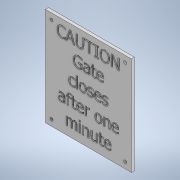
# Autodesk Inventor part: warningSignV2
Saved by Autodesk Inventor 2021.2 (Build 252289000, 289)
## iProperties
Created: 2020-11-24
Part Number: warningSignV2
Material: Generic
Document SubType Name: Modeling
Designer: robst
Density: 1 g/cm^3
Appearance: Default
Author: robst
Autodesk Inventor part; units mm, degrees
ref_plane "YZ Plane" through (0, 0, 0) normal (1, 0, 0) x (0, 1, 0)
ref_plane "XZ Plane" through (0, 0, 0) normal (0, 1, 0) x (-1, 0, 0)
ref_plane "XY Plane" through (0, 0, 0) normal (0, 0, 1) x (1, 0, 0)
sketch "Sketch4" plane through (0, 0, 0) normal (0, 0, 1) x (1, 0, 0)
  line L0 (-88.9, -101.6) -> (88.9, -101.6)
  line L1 (88.9, -101.6) -> (88.9, 101.6)
  line L2 (88.9, 101.6) -> (-88.9, 101.6)
  line L3 (-88.9, 101.6) -> (-88.9, -101.6)
  line L4 (-88.9, -101.6) -> (88.9, 101.6) construction
  line L5 (88.9, -101.6) -> (-88.9, 101.6) construction
  point P0 (0, 0)
  dimension "d12" = 203.2
  dimension "d13" = 177.8
  constraints: 12 end point, 2 midpoint, 2 parallel, 1 horizontal, 1 perpendicular
  measures "d12" distance of L2.end L0.start
  measures "d13" distance of L0.start L0.end
extrude "Extrusion2" add sketch "Sketch4" against normal blind 6.35
sketch "Sketch5" plane through (0, 0, 0) normal (0, 0, 1) x (1, 0, 0)
  line L0 (-88.9, -101.6) -> (-88.9, 101.6) construction
  line L1 (-88.9, 67.31) -> (88.9, 67.31) construction
  line L2 (88.9, 101.6) -> (88.9, -101.6) construction
  line L3 (88.9, 101.6) -> (-88.9, 101.6) construction
  spline S0 degree 2 poles (-54.5935, 66.9024) (-56.8165, 66.9024) (-60.5771, 68.403) (-61.948, 69.9035) knots 0 0 0 1 2 2 2
  spline S1 degree 2 poles (-61.948, 69.9035) (-63.3189, 71.3855) (-64.8194, 75.8316) (-64.8194, 78.7215) knots 0 0 0 1 2 2 2
  spline S2 degree 2 poles (-64.8194, 78.7215) (-64.8194, 81.5929) (-63.3559, 85.8536) (-61.9665, 87.4283) knots 0 0 0 1 2 2 2
  spline S3 degree 2 poles (-61.9665, 87.4283) (-60.5957, 88.9659) (-56.8536, 90.5776) (-54.538, 90.5776) knots 0 0 0 1 2 2 2
  spline S4 degree 2 poles (-54.538, 90.5776) (-53.3894, 90.5776) (-51.3702, 90.2441) (-50.518, 89.9847) knots 0 0 0 1 2 2 2
  spline S5 degree 2 poles (-50.518, 89.9847) (-49.777, 89.7439) (-48.2394, 89.0585) (-47.4799, 88.6509) knots 0 0 0 1 2 2 2
  line L4 (-47.4799, 88.6509) -> (-47.4799, 84.983)
  line L5 (-47.4799, 84.983) -> (-47.7207, 84.983)
  spline S6 degree 2 poles (-47.7207, 84.983) (-48.1283, 85.3535) (-49.388, 86.3909) (-50.2957, 86.8911) knots 0 0 0 1 2 2 2
  spline S7 degree 2 poles (-50.2957, 86.8911) (-51.1664, 87.3727) (-53.2227, 87.984) (-54.5565, 87.984) knots 0 0 0 1 2 2 2
  spline S8 degree 2 poles (-54.5565, 87.984) (-56.02, 87.984) (-58.632, 86.7799) (-59.6138, 85.6313) knots 0 0 0 1 2 2 2
  spline S9 degree 2 poles (-59.6138, 85.6313) (-60.5771, 84.4643) (-61.6516, 80.926) (-61.6516, 78.7215) knots 0 0 0 1 2 2 2
  spline S10 degree 2 poles (-61.6516, 78.7215) (-61.6516, 76.3688) (-60.5216, 72.9787) (-59.5397, 71.8116) knots 0 0 0 1 2 2 2
  spline S11 degree 2 poles (-59.5397, 71.8116) (-58.5764, 70.6816) (-56.0014, 69.533) (-54.5565, 69.533) knots 0 0 0 1 2 2 2
  spline S12 degree 2 poles (-54.5565, 69.533) (-53.2412, 69.533) (-50.9997, 70.1814) (-50.129, 70.663) knots 0 0 0 1 2 2 2
  spline S13 degree 2 poles (-50.129, 70.663) (-49.2953, 71.1447) (-48.0542, 72.1451) (-47.7022, 72.497) knots 0 0 0 1 2 2 2
  line L6 (-47.7022, 72.497) -> (-47.4799, 72.497)
  line L7 (-47.4799, 72.497) -> (-47.4799, 68.8661)
  spline S14 degree 2 poles (-47.4799, 68.8661) (-48.2394, 68.5141) (-49.5732, 67.8658) (-50.518, 67.5694) knots 0 0 0 1 2 2 2
  spline S15 degree 2 poles (-50.518, 67.5694) (-51.5184, 67.2359) (-53.2227, 66.9024) (-54.5935, 66.9024) knots 0 0 0 1 2 2 2
  line L8 (-47.1094, 67.31) -> (-39.4029, 90.17)
  line L9 (-39.4029, 90.17) -> (-35.6609, 90.17)
  line L10 (-35.6609, 90.17) -> (-27.9544, 67.31)
  line L11 (-27.9544, 67.31) -> (-31.1593, 67.31)
  line L12 (-31.1593, 67.31) -> (-33.2341, 73.7012)
  line L13 (-33.2341, 73.7012) -> (-41.9594, 73.7012)
  line L14 (-41.9594, 73.7012) -> (-44.0342, 67.31)
  line L15 (-44.0342, 67.31) -> (-47.1094, 67.31)
  line L16 (-34.0677, 76.2947) -> (-37.606, 87.0578)
  line L17 (-37.606, 87.0578) -> (-41.1258, 76.2947)
  line L18 (-41.1258, 76.2947) -> (-34.0677, 76.2947)
  spline S16 degree 2 poles (-17.5062, 66.8283) (-19.5255, 66.8283) (-22.5265, 67.8843) (-23.5825, 68.9402) knots 0 0 0 1 2 2 2
  spline S17 degree 2 poles (-23.5825, 68.9402) (-24.7866, 70.1258) (-25.7684, 73.4603) (-25.7684, 75.9057) knots 0 0 0 1 2 2 2
  line L19 (-25.7684, 75.9057) -> (-25.7684, 90.17)
  line L20 (-25.7684, 90.17) -> (-22.7303, 90.17)
  line L21 (-22.7303, 90.17) -> (-22.7303, 75.9057)
  spline S18 degree 2 poles (-22.7303, 75.9057) (-22.7303, 74.3125) (-22.3228, 72.1636) (-21.7485, 71.2929) knots 0 0 0 1 2 2 2
  spline S19 degree 2 poles (-21.7485, 71.2929) (-21.1372, 70.3666) (-19.0253, 69.4219) (-17.5062, 69.4219) knots 0 0 0 1 2 2 2
  spline S20 degree 2 poles (-17.5062, 69.4219) (-16.0798, 69.4219) (-13.8568, 70.3666) (-13.2455, 71.2929) knots 0 0 0 1 2 2 2
  spline S21 degree 2 poles (-13.2455, 71.2929) (-12.6712, 72.1636) (-12.2636, 74.294) (-12.2636, 75.8316) knots 0 0 0 1 2 2 2
  line L22 (-12.2636, 75.8316) -> (-12.2636, 90.17)
  line L23 (-12.2636, 90.17) -> (-9.2255, 90.17)
  line L24 (-9.2255, 90.17) -> (-9.2255, 75.9057)
  spline S22 degree 2 poles (-9.2255, 75.9057) (-9.2255, 73.5159) (-10.1888, 70.1073) (-11.4115, 68.9402) knots 0 0 0 1 2 2 2
  spline S23 degree 2 poles (-11.4115, 68.9402) (-12.5045, 67.8658) (-15.3944, 66.8283) (-17.5062, 66.8283) knots 0 0 0 1 2 2 2
  line L25 (0.4631, 67.31) -> (0.4631, 87.4653)
  line L26 (0.4631, 87.4653) -> (-7.2063, 87.4653)
  line L27 (-7.2063, 87.4653) -> (-7.2063, 90.17)
  line L28 (-7.2063, 90.17) -> (11.1706, 90.17)
  line L29 (11.1706, 90.17) -> (11.1706, 87.4653)
  line L30 (11.1706, 87.4653) -> (3.5012, 87.4653)
  line L31 (3.5012, 87.4653) -> (3.5012, 67.31)
  line L32 (3.5012, 67.31) -> (0.4631, 67.31)
  line L33 (21.4706, 67.31) -> (12.6156, 67.31)
  line L34 (12.6156, 67.31) -> (12.6156, 69.6442)
  line L35 (12.6156, 69.6442) -> (15.5241, 69.6442)
  line L36 (15.5241, 69.6442) -> (15.5241, 87.8358)
  line L37 (15.5241, 87.8358) -> (12.6156, 87.8358)
  line L38 (12.6156, 87.8358) -> (12.6156, 90.17)
  line L39 (12.6156, 90.17) -> (21.4706, 90.17)
  line L40 (21.4706, 90.17) -> (21.4706, 87.8358)
  line L41 (21.4706, 87.8358) -> (18.5622, 87.8358)
  line L42 (18.5622, 87.8358) -> (18.5622, 69.6442)
  line L43 (18.5622, 69.6442) -> (21.4706, 69.6442)
  line L44 (21.4706, 69.6442) -> (21.4706, 67.31)
  spline S24 degree 2 poles (41.4036, 87.558) (42.7004, 86.0389) (44.1454, 81.5929) (44.1454, 78.74) knots 0 0 0 1 2 2 2
  spline S25 degree 2 poles (44.1454, 78.74) (44.1454, 75.9612) (42.7375, 71.4596) (41.4036, 69.9406) knots 0 0 0 1 2 2 2
  spline S26 degree 2 poles (41.4036, 69.9406) (39.9957, 68.3474) (36.2722, 66.8283) (34.0306, 66.8283) knots 0 0 0 1 2 2 2
  spline S27 degree 2 poles (34.0306, 66.8283) (31.715, 66.8283) (28.01, 68.403) (26.6577, 69.9406) knots 0 0 0 1 2 2 2
  spline S28 degree 2 poles (26.6577, 69.9406) (25.3424, 71.4596) (23.9345, 75.9242) (23.9345, 78.74) knots 0 0 0 1 2 2 2
  spline S29 degree 2 poles (23.9345, 78.74) (23.9345, 81.6114) (25.3609, 85.9833) (26.6762, 87.558) knots 0 0 0 1 2 2 2
  spline S30 degree 2 poles (26.6762, 87.558) (28.01, 89.077) (31.7335, 90.6517) (34.0306, 90.6517) knots 0 0 0 1 2 2 2
  spline S31 degree 2 poles (34.0306, 90.6517) (36.3648, 90.6517) (40.1069, 89.0214) (41.4036, 87.558) knots 0 0 0 1 2 2 2
  spline S32 degree 2 poles (40.9776, 78.74) (40.9776, 81.0001) (39.9957, 84.5013) (39.1065, 85.6499) knots 0 0 0 1 2 2 2
  spline S33 degree 2 poles (39.1065, 85.6499) (38.1988, 86.8355) (35.6423, 88.0211) (34.0492, 88.0211) knots 0 0 0 1 2 2 2
  spline S34 degree 2 poles (34.0492, 88.0211) (32.4004, 88.0211) (29.9181, 86.8725) (28.9733, 85.6499) knots 0 0 0 1 2 2 2
  spline S35 degree 2 poles (28.9733, 85.6499) (28.0656, 84.4828) (27.1023, 80.963) (27.1023, 78.74) knots 0 0 0 1 2 2 2
  spline S36 degree 2 poles (27.1023, 78.74) (27.1023, 74.2384) (30.8814, 69.4589) (34.0492, 69.4589) knots 0 0 0 1 2 2 2
  spline S37 degree 2 poles (34.0492, 69.4589) (37.217, 69.4589) (40.9776, 74.2384) (40.9776, 78.74) knots 0 0 0 1 2 2 2
  line L45 (63.8376, 67.31) -> (60.4289, 67.31)
  line L46 (60.4289, 67.31) -> (50.3142, 87.0207)
  line L47 (50.3142, 87.0207) -> (50.3142, 67.31)
  line L48 (50.3142, 67.31) -> (47.4799, 67.31)
  line L49 (47.4799, 67.31) -> (47.4799, 90.17)
  line L50 (47.4799, 90.17) -> (51.7962, 90.17)
  line L51 (51.7962, 90.17) -> (61.0032, 72.071)
  line L52 (61.0032, 72.071) -> (61.0032, 90.17)
  line L53 (61.0032, 90.17) -> (63.8376, 90.17)
  line L54 (63.8376, 90.17) -> (63.8376, 67.31)
  spline S38 degree 2 poles (-20.3869, 29.1894) (-22.8137, 29.1894) (-26.8336, 30.6714) (-28.2786, 32.172) knots 0 0 0 1 2 2 2
  spline S39 degree 2 poles (-28.2786, 32.172) (-29.7236, 33.691) (-31.2611, 38.1741) (-31.2611, 41.0826) knots 0 0 0 1 2 2 2
  spline S40 degree 2 poles (-31.2611, 41.0826) (-31.2611, 43.8428) (-29.705, 48.2147) (-28.2601, 49.7708) knots 0 0 0 1 2 2 2
  spline S41 degree 2 poles (-28.2601, 49.7708) (-26.8707, 51.2714) (-22.7952, 52.9016) (-20.3684, 52.9016) knots 0 0 0 1 2 2 2
  spline S42 degree 2 poles (-20.3684, 52.9016) (-19.2013, 52.9016) (-17.0894, 52.5681) (-16.1261, 52.2717) knots 0 0 0 1 2 2 2
  spline S43 degree 2 poles (-16.1261, 52.2717) (-15.3481, 52.0494) (-13.4585, 51.2343) (-12.8842, 50.9379) knots 0 0 0 1 2 2 2
  line L55 (-12.8842, 50.9379) -> (-12.8842, 47.2699)
  line L56 (-12.8842, 47.2699) -> (-13.1436, 47.2699)
  spline S44 degree 2 poles (-13.1436, 47.2699) (-13.7179, 47.7701) (-14.922, 48.6779) (-16.0335, 49.1966) knots 0 0 0 1 2 2 2
  spline S45 degree 2 poles (-16.0335, 49.1966) (-16.9597, 49.6597) (-19.3495, 50.271) (-20.7203, 50.271) knots 0 0 0 1 2 2 2
  spline S46 degree 2 poles (-20.7203, 50.271) (-24.0178, 50.271) (-28.0933, 45.3063) (-28.0933, 41.1752) knots 0 0 0 1 2 2 2
  spline S47 degree 2 poles (-28.0933, 41.1752) (-28.0933, 38.8781) (-27.0189, 35.4324) (-26, 34.2468) knots 0 0 0 1 2 2 2
  spline S48 degree 2 poles (-26, 34.2468) (-25.0182, 33.0612) (-22.2394, 31.82) (-20.498, 31.82) knots 0 0 0 1 2 2 2
  spline S49 degree 2 poles (-20.498, 31.82) (-19.2198, 31.82) (-16.6633, 32.1905) (-15.7927, 32.561) knots 0 0 0 1 2 2 2
  line L57 (-15.7927, 32.561) -> (-15.7927, 38.4705)
  line L58 (-15.7927, 38.4705) -> (-21.0908, 38.4705)
  line L59 (-21.0908, 38.4705) -> (-21.0908, 41.1381)
  line L60 (-21.0908, 41.1381) -> (-12.7916, 41.1381)
  line L61 (-12.7916, 41.1381) -> (-12.7916, 31.1531)
  spline S50 degree 2 poles (-12.7916, 31.1531) (-13.3659, 30.8937) (-15.3295, 30.0972) (-16.1632, 29.8563) knots 0 0 0 1 2 2 2
  spline S51 degree 2 poles (-16.1632, 29.8563) (-17.2932, 29.5229) (-19.1087, 29.1894) (-20.3869, 29.1894) knots 0 0 0 1 2 2 2
  spline S52 degree 2 poles (0.3612, 31.4495) (0.0093, 31.1901) (-1.1763, 30.2639) (-1.7321, 29.986) knots 0 0 0 1 2 2 2
  spline S53 degree 2 poles (-1.7321, 29.986) (-2.4916, 29.5785) (-3.9181, 29.1524) (-5.2148, 29.1524) knots 0 0 0 1 2 2 2
  spline S54 degree 2 poles (-5.2148, 29.1524) (-6.2708, 29.1524) (-8.1788, 29.949) (-8.9013, 30.6714) knots 0 0 0 1 2 2 2
  spline S55 degree 2 poles (-8.9013, 30.6714) (-9.5867, 31.3754) (-10.4204, 33.4502) (-10.4204, 34.5988) knots 0 0 0 1 2 2 2
  spline S56 degree 2 poles (-10.4204, 34.5988) (-10.4204, 36.3772) (-8.9198, 38.8966) (-7.2896, 39.6191) knots 0 0 0 1 2 2 2
  spline S57 degree 2 poles (-7.2896, 39.6191) (-5.8447, 40.286) (-1.9173, 40.7862) (0.3612, 40.9158) knots 0 0 0 1 2 2 2
  line L62 (0.3612, 40.9158) -> (0.3612, 41.4716)
  spline S58 degree 2 poles (0.3612, 41.4716) (0.3612, 42.4719) (-0.2501, 43.7131) (-0.8058, 44.0651) knots 0 0 0 1 2 2 2
  spline S59 degree 2 poles (-0.8058, 44.0651) (-1.3616, 44.4171) (-2.9548, 44.6394) (-3.8069, 44.6394) knots 0 0 0 1 2 2 2
  spline S60 degree 2 poles (-3.8069, 44.6394) (-4.8073, 44.6394) (-7.5119, 44.0466) (-8.8643, 43.4723) knots 0 0 0 1 2 2 2
  line L63 (-8.8643, 43.4723) -> (-9.031, 43.4723)
  line L64 (-9.031, 43.4723) -> (-9.031, 46.4178)
  spline S61 degree 2 poles (-9.031, 46.4178) (-8.2344, 46.6401) (-5.2519, 47.1958) (-3.7884, 47.1958) knots 0 0 0 1 2 2 2
  spline S62 degree 2 poles (-3.7884, 47.1958) (-2.01, 47.1958) (0.4168, 46.6401) (1.3801, 45.9176) knots 0 0 0 1 2 2 2
  spline S63 degree 2 poles (1.3801, 45.9176) (2.3249, 45.2137) (3.2512, 42.9721) (3.2512, 41.3604) knots 0 0 0 1 2 2 2
  line L65 (3.2512, 41.3604) -> (3.2512, 29.634)
  line L66 (3.2512, 29.634) -> (0.3612, 29.634)
  line L67 (0.3612, 29.634) -> (0.3612, 31.4495)
  line L68 (0.3612, 33.8578) -> (0.3612, 38.6187)
  spline S64 degree 2 poles (0.3612, 38.6187) (-0.6762, 38.5261) (-3.8069, 38.2112) (-4.7887, 37.9148) knots 0 0 0 1 2 2 2
  spline S65 degree 2 poles (-4.7887, 37.9148) (-5.9373, 37.5628) (-7.4378, 36.0993) (-7.4378, 34.8025) knots 0 0 0 1 2 2 2
  spline S66 degree 2 poles (-7.4378, 34.8025) (-7.4378, 33.3205) (-5.7706, 31.82) (-4.1774, 31.82) knots 0 0 0 1 2 2 2
  spline S67 degree 2 poles (-4.1774, 31.82) (-2.8251, 31.82) (-0.6021, 32.9871) (0.3612, 33.8578) knots 0 0 0 1 2 2 2
  spline S68 degree 2 poles (12.4952, 29.3006) (10.1425, 29.3006) (7.4934, 31.9867) (7.4934, 34.8952) knots 0 0 0 1 2 2 2
  line L69 (7.4934, 34.8952) -> (7.4934, 44.3985)
  line L70 (7.4934, 44.3985) -> (5.5483, 44.3985)
  line L71 (5.5483, 44.3985) -> (5.5483, 46.7883)
  line L72 (5.5483, 46.7883) -> (7.4934, 46.7883)
  line L73 (7.4934, 46.7883) -> (7.4934, 51.716)
  line L74 (7.4934, 51.716) -> (10.3833, 51.716)
  line L75 (10.3833, 51.716) -> (10.3833, 46.7883)
  line L76 (10.3833, 46.7883) -> (15.7, 46.7883)
  line L77 (15.7, 46.7883) -> (15.7, 44.3985)
  line L78 (15.7, 44.3985) -> (10.3833, 44.3985)
  line L79 (10.3833, 44.3985) -> (10.3833, 36.229)
  spline S69 degree 2 poles (10.3833, 36.229) (10.3833, 34.9322) (10.476, 33.5058) (10.7909, 32.8944) knots 0 0 0 1 2 2 2
  spline S70 degree 2 poles (10.7909, 32.8944) (11.0502, 32.3572) (12.2173, 31.82) (13.2177, 31.82) knots 0 0 0 1 2 2 2
  spline S71 degree 2 poles (13.2177, 31.82) (13.9216, 31.82) (15.2369, 32.2461) (15.5333, 32.3757) knots 0 0 0 1 2 2 2
  line L80 (15.5333, 32.3757) -> (15.7, 32.3757)
  line L81 (15.7, 32.3757) -> (15.7, 29.7822)
  spline S72 degree 2 poles (15.7, 29.7822) (14.8849, 29.5599) (13.2177, 29.3006) (12.4952, 29.3006) knots 0 0 0 1 2 2 2
  spline S73 degree 2 poles (25.2775, 29.245) (21.165, 29.245) (16.6448, 33.8578) (16.6448, 38.1185) knots 0 0 0 1 2 2 2
  spline S74 degree 2 poles (16.6448, 38.1185) (16.6448, 42.3052) (21.0353, 47.2699) (24.5736, 47.2699) knots 0 0 0 1 2 2 2
  spline S75 degree 2 poles (24.5736, 47.2699) (26.1667, 47.2699) (28.6306, 46.3437) (29.5383, 45.3619) knots 0 0 0 1 2 2 2
  spline S76 degree 2 poles (29.5383, 45.3619) (30.4646, 44.38) (31.4464, 41.5457) (31.4464, 39.4894) knots 0 0 0 1 2 2 2
  line L82 (31.4464, 39.4894) -> (31.4464, 37.9148)
  line L83 (31.4464, 37.9148) -> (19.5718, 37.9148)
  spline S77 degree 2 poles (19.5718, 37.9148) (19.5718, 34.9322) (22.5729, 31.7644) (25.2405, 31.7644) knots 0 0 0 1 2 2 2
  spline S78 degree 2 poles (25.2405, 31.7644) (26.1853, 31.7644) (28.0192, 32.1905) (28.7603, 32.5239) knots 0 0 0 1 2 2 2
  spline S79 degree 2 poles (28.7603, 32.5239) (29.5383, 32.8944) (30.6128, 33.5428) (30.9647, 33.8392) knots 0 0 0 1 2 2 2
  line L84 (30.9647, 33.8392) -> (31.1315, 33.8392)
  line L85 (31.1315, 33.8392) -> (31.1315, 30.69)
  spline S80 degree 2 poles (31.1315, 30.69) (30.6313, 30.4862) (29.1122, 29.8934) (28.5194, 29.7267) knots 0 0 0 1 2 2 2
  spline S81 degree 2 poles (28.5194, 29.7267) (27.6858, 29.4858) (26.3149, 29.245) (25.2775, 29.245) knots 0 0 0 1 2 2 2
  spline S82 degree 2 poles (28.6306, 40.1192) (28.5935, 41.2863) (28.1119, 42.9906) (27.6487, 43.5649) knots 0 0 0 1 2 2 2
  spline S83 degree 2 poles (27.6487, 43.5649) (27.1486, 44.2133) (25.5739, 44.8987) (24.4068, 44.8987) knots 0 0 0 1 2 2 2
  spline S84 degree 2 poles (24.4068, 44.8987) (23.2583, 44.8987) (21.6466, 44.2133) (20.9797, 43.5464) knots 0 0 0 1 2 2 2
  spline S85 degree 2 poles (20.9797, 43.5464) (20.3313, 42.861) (19.6644, 41.2122) (19.5718, 40.1192) knots 0 0 0 1 2 2 2
  line L86 (19.5718, 40.1192) -> (28.6306, 40.1192)
  spline S86 degree 2 poles (-32.7617, -9.0423) (-34.5401, -9.0423) (-37.4856, -7.9493) (-38.5415, -6.8378) knots 0 0 0 1 2 2 2
  spline S87 degree 2 poles (-38.5415, -6.8378) (-39.5974, -5.7448) (-40.7645, -2.3733) (-40.7645, -0.1132) knots 0 0 0 1 2 2 2
  spline S88 degree 2 poles (-40.7645, -0.1132) (-40.7645, 2.1469) (-39.5604, 5.4443) (-38.5415, 6.5559) knots 0 0 0 1 2 2 2
  spline S89 degree 2 poles (-38.5415, 6.5559) (-37.5226, 7.6859) (-34.503, 8.89) (-32.7617, 8.89) knots 0 0 0 1 2 2 2
  spline S90 degree 2 poles (-32.7617, 8.89) (-31.3538, 8.89) (-28.7232, 8.0934) (-27.7043, 7.5747) knots 0 0 0 1 2 2 2
  line L87 (-27.7043, 7.5747) -> (-27.7043, 4.3328)
  line L88 (-27.7043, 4.3328) -> (-27.871, 4.3328)
  spline S91 degree 2 poles (-27.871, 4.3328) (-28.186, 4.5922) (-29.1493, 5.2591) (-29.8347, 5.6111) knots 0 0 0 1 2 2 2
  spline S92 degree 2 poles (-29.8347, 5.6111) (-30.446, 5.9075) (-32.0762, 6.3706) (-32.8173, 6.3706) knots 0 0 0 1 2 2 2
  spline S93 degree 2 poles (-32.8173, 6.3706) (-35.0588, 6.3706) (-37.782, 2.9805) (-37.782, -0.1132) knots 0 0 0 1 2 2 2
  spline S94 degree 2 poles (-37.782, -0.1132) (-37.782, -3.1328) (-35.1514, -6.5229) (-32.8173, -6.5229) knots 0 0 0 1 2 2 2
  spline S95 degree 2 poles (-32.8173, -6.5229) (-31.4093, -6.5229) (-28.8529, -5.3558) (-27.871, -4.4481) knots 0 0 0 1 2 2 2
  line L89 (-27.871, -4.4481) -> (-27.7043, -4.4481)
  line L90 (-27.7043, -4.4481) -> (-27.7043, -7.69)
  spline S96 degree 2 poles (-27.7043, -7.69) (-28.1304, -7.8937) (-29.4272, -8.468) (-29.9459, -8.5977) knots 0 0 0 1 2 2 2
  spline S97 degree 2 poles (-29.9459, -8.5977) (-30.6869, -8.82) (-31.8539, -9.0423) (-32.7617, -9.0423) knots 0 0 0 1 2 2 2
  line L91 (-22.1283, -8.6533) -> (-25.0182, -8.6533)
  line L92 (-25.0182, -8.6533) -> (-25.0182, 15.2256)
  line L93 (-25.0182, 15.2256) -> (-22.1283, 15.2256)
  line L94 (-22.1283, 15.2256) -> (-22.1283, -8.6533)
  spline S98 degree 2 poles (-3.7884, -0.0761) (-3.7884, -4.411) (-7.9565, -9.1349) (-11.4393, -9.1349) knots 0 0 0 1 2 2 2
  spline S99 degree 2 poles (-11.4393, -9.1349) (-15.0146, -9.1349) (-19.1087, -4.2628) (-19.1087, -0.0761) knots 0 0 0 1 2 2 2
  spline S100 degree 2 poles (-19.1087, -0.0761) (-19.1087, 4.2217) (-14.8849, 8.9826) (-11.4393, 8.9826) knots 0 0 0 1 2 2 2
  spline S101 degree 2 poles (-11.4393, 8.9826) (-7.9565, 8.9826) (-3.7884, 4.2402) (-3.7884, -0.0761) knots 0 0 0 1 2 2 2
  spline S102 degree 2 poles (-6.7709, -0.0761) (-6.7709, 3.2584) (-9.1977, 6.5003) (-11.4393, 6.5003) knots 0 0 0 1 2 2 2
  spline S103 degree 2 poles (-11.4393, 6.5003) (-13.6808, 6.5003) (-16.1261, 3.2584) (-16.1261, -0.0761) knots 0 0 0 1 2 2 2
  spline S104 degree 2 poles (-16.1261, -0.0761) (-16.1261, -3.318) (-13.6808, -6.6526) (-11.4393, -6.6526) knots 0 0 0 1 2 2 2
  spline S105 degree 2 poles (-11.4393, -6.6526) (-9.2162, -6.6526) (-6.7709, -3.3736) (-6.7709, -0.0761) knots 0 0 0 1 2 2 2
  spline S106 degree 2 poles (3.8069, -9.0608) (2.0841, -9.0608) (-0.8985, -8.1346) (-1.8803, -7.6159) knots 0 0 0 1 2 2 2
  line L95 (-1.8803, -7.6159) -> (-1.8803, -4.374)
  line L96 (-1.8803, -4.374) -> (-1.7321, -4.374)
  spline S107 degree 2 poles (-1.7321, -4.374) (-1.3616, -4.6704) (-0.3612, -5.3743) (0.4724, -5.7634) knots 0 0 0 1 2 2 2
  spline S108 degree 2 poles (0.4724, -5.7634) (1.1949, -6.1153) (2.9733, -6.634) (3.9181, -6.634) knots 0 0 0 1 2 2 2
  spline S109 degree 2 poles (3.9181, -6.634) (4.6035, -6.634) (6.1781, -6.3191) (6.5486, -6.0598) knots 0 0 0 1 2 2 2
  spline S110 degree 2 poles (6.5486, -6.0598) (7.0859, -5.7078) (7.5675, -4.9112) (7.5675, -4.0961) knots 0 0 0 1 2 2 2
  spline S111 degree 2 poles (7.5675, -4.0961) (7.5675, -3.0772) (6.456, -2.0213) (5.0296, -1.6693) knots 0 0 0 1 2 2 2
  spline S112 degree 2 poles (5.0296, -1.6693) (4.4738, -1.5396) (2.6954, -1.1691) (1.9359, -0.9653) knots 0 0 0 1 2 2 2
  spline S113 degree 2 poles (1.9359, -0.9653) (-0.0278, -0.3911) (-1.8062, 1.9801) (-1.8062, 3.6659) knots 0 0 0 1 2 2 2
  spline S114 degree 2 poles (-1.8062, 3.6659) (-1.8062, 6.0001) (1.695, 8.9085) (4.585, 8.9085) knots 0 0 0 1 2 2 2
  spline S115 degree 2 poles (4.585, 8.9085) (6.0114, 8.9085) (8.9013, 8.2046) (9.8832, 7.6674) knots 0 0 0 1 2 2 2
  line L97 (9.8832, 7.6674) -> (9.8832, 4.5737)
  line L98 (9.8832, 4.5737) -> (9.735, 4.5737)
  spline S116 degree 2 poles (9.735, 4.5737) (8.6234, 5.4629) (5.9188, 6.4818) (4.5294, 6.4818) knots 0 0 0 1 2 2 2
  spline S117 degree 2 poles (4.5294, 6.4818) (3.103, 6.4818) (1.1393, 5.2776) (1.1393, 4.0735) knots 0 0 0 1 2 2 2
  spline S118 degree 2 poles (1.1393, 4.0735) (1.1393, 2.9805) (2.3064, 1.9246) (3.6031, 1.5911) knots 0 0 0 1 2 2 2
  spline S119 degree 2 poles (3.6031, 1.5911) (4.233, 1.4244) (5.8262, 1.0909) (6.6968, 0.8872) knots 0 0 0 1 2 2 2
  spline S120 degree 2 poles (6.6968, 0.8872) (8.5864, 0.4055) (10.513, -1.799) (10.513, -3.7071) knots 0 0 0 1 2 2 2
  spline S121 degree 2 poles (10.513, -3.7071) (10.513, -4.8186) (9.6423, -6.7822) (8.7902, -7.5047) knots 0 0 0 1 2 2 2
  spline S122 degree 2 poles (8.7902, -7.5047) (7.8824, -8.2642) (5.5668, -9.0608) (3.8069, -9.0608) knots 0 0 0 1 2 2 2
  spline S123 degree 2 poles (20.6462, -9.0423) (16.5337, -9.0423) (12.0135, -4.4295) (12.0135, -0.1688) knots 0 0 0 1 2 2 2
  spline S124 degree 2 poles (12.0135, -0.1688) (12.0135, 4.0179) (16.404, 8.9826) (19.9423, 8.9826) knots 0 0 0 1 2 2 2
  spline S125 degree 2 poles (19.9423, 8.9826) (21.5355, 8.9826) (23.9993, 8.0564) (24.907, 7.0746) knots 0 0 0 1 2 2 2
  spline S126 degree 2 poles (24.907, 7.0746) (25.8333, 6.0927) (26.8151, 3.2584) (26.8151, 1.2021) knots 0 0 0 1 2 2 2
  line L99 (26.8151, 1.2021) -> (26.8151, -0.3725)
  line L100 (26.8151, -0.3725) -> (14.9405, -0.3725)
  spline S127 degree 2 poles (14.9405, -0.3725) (14.9405, -3.3551) (17.9416, -6.5229) (20.6092, -6.5229) knots 0 0 0 1 2 2 2
  spline S128 degree 2 poles (20.6092, -6.5229) (21.554, -6.5229) (23.388, -6.0968) (24.129, -5.7634) knots 0 0 0 1 2 2 2
  spline S129 degree 2 poles (24.129, -5.7634) (24.907, -5.3929) (25.9815, -4.7445) (26.3335, -4.4481) knots 0 0 0 1 2 2 2
  line L101 (26.3335, -4.4481) -> (26.5002, -4.4481)
  line L102 (26.5002, -4.4481) -> (26.5002, -7.5973)
  spline S130 degree 2 poles (26.5002, -7.5973) (26, -7.8011) (24.4809, -8.3939) (23.8881, -8.5606) knots 0 0 0 1 2 2 2
  spline S131 degree 2 poles (23.8881, -8.5606) (23.0545, -8.8015) (21.6837, -9.0423) (20.6462, -9.0423) knots 0 0 0 1 2 2 2
  spline S132 degree 2 poles (23.9993, 1.8319) (23.9622, 2.999) (23.4806, 4.7033) (23.0175, 5.2776) knots 0 0 0 1 2 2 2
  spline S133 degree 2 poles (23.0175, 5.2776) (22.5173, 5.926) (20.9427, 6.6114) (19.7756, 6.6114) knots 0 0 0 1 2 2 2
  spline S134 degree 2 poles (19.7756, 6.6114) (18.627, 6.6114) (17.0153, 5.926) (16.3484, 5.2591) knots 0 0 0 1 2 2 2
  spline S135 degree 2 poles (16.3484, 5.2591) (15.7, 4.5737) (15.0331, 2.9249) (14.9405, 1.8319) knots 0 0 0 1 2 2 2
  line L103 (14.9405, 1.8319) -> (23.9993, 1.8319)
  spline S136 degree 2 poles (34.3734, -9.0608) (32.6505, -9.0608) (29.668, -8.1346) (28.6862, -7.6159) knots 0 0 0 1 2 2 2
  line L104 (28.6862, -7.6159) -> (28.6862, -4.374)
  line L105 (28.6862, -4.374) -> (28.8344, -4.374)
  spline S137 degree 2 poles (28.8344, -4.374) (29.2049, -4.6704) (30.2052, -5.3743) (31.0388, -5.7634) knots 0 0 0 1 2 2 2
  spline S138 degree 2 poles (31.0388, -5.7634) (31.7613, -6.1153) (33.5397, -6.634) (34.4845, -6.634) knots 0 0 0 1 2 2 2
  spline S139 degree 2 poles (34.4845, -6.634) (35.1699, -6.634) (36.7446, -6.3191) (37.1151, -6.0598) knots 0 0 0 1 2 2 2
  spline S140 degree 2 poles (37.1151, -6.0598) (37.6523, -5.7078) (38.134, -4.9112) (38.134, -4.0961) knots 0 0 0 1 2 2 2
  spline S141 degree 2 poles (38.134, -4.0961) (38.134, -3.0772) (37.0225, -2.0213) (35.596, -1.6693) knots 0 0 0 1 2 2 2
  spline S142 degree 2 poles (35.596, -1.6693) (35.0403, -1.5396) (33.2619, -1.1691) (32.5023, -0.9653) knots 0 0 0 1 2 2 2
  spline S143 degree 2 poles (32.5023, -0.9653) (30.5387, -0.3911) (28.7603, 1.9801) (28.7603, 3.6659) knots 0 0 0 1 2 2 2
  spline S144 degree 2 poles (28.7603, 3.6659) (28.7603, 6.0001) (32.2615, 8.9085) (35.1514, 8.9085) knots 0 0 0 1 2 2 2
  spline S145 degree 2 poles (35.1514, 8.9085) (36.5779, 8.9085) (39.4678, 8.2046) (40.4496, 7.6674) knots 0 0 0 1 2 2 2
  line L106 (40.4496, 7.6674) -> (40.4496, 4.5737)
  line L107 (40.4496, 4.5737) -> (40.3014, 4.5737)
  spline S146 degree 2 poles (40.3014, 4.5737) (39.1899, 5.4629) (36.4852, 6.4818) (35.0958, 6.4818) knots 0 0 0 1 2 2 2
  spline S147 degree 2 poles (35.0958, 6.4818) (33.6694, 6.4818) (31.7057, 5.2776) (31.7057, 4.0735) knots 0 0 0 1 2 2 2
  spline S148 degree 2 poles (31.7057, 4.0735) (31.7057, 2.9805) (32.8728, 1.9246) (34.1696, 1.5911) knots 0 0 0 1 2 2 2
  spline S149 degree 2 poles (34.1696, 1.5911) (34.7994, 1.4244) (36.3926, 1.0909) (37.2633, 0.8872) knots 0 0 0 1 2 2 2
  spline S150 degree 2 poles (37.2633, 0.8872) (39.1528, 0.4055) (41.0795, -1.799) (41.0795, -3.7071) knots 0 0 0 1 2 2 2
  spline S151 degree 2 poles (41.0795, -3.7071) (41.0795, -4.8186) (40.2088, -6.7822) (39.3566, -7.5047) knots 0 0 0 1 2 2 2
  spline S152 degree 2 poles (39.3566, -7.5047) (38.4489, -8.2642) (36.1333, -9.0608) (34.3734, -9.0608) knots 0 0 0 1 2 2 2
  spline S153 degree 2 poles (-51.2775, -45.2733) (-51.6295, -45.5327) (-52.8151, -46.4589) (-53.3709, -46.7368) knots 0 0 0 1 2 2 2
  spline S154 degree 2 poles (-53.3709, -46.7368) (-54.1304, -47.1444) (-55.5568, -47.5704) (-56.8536, -47.5704) knots 0 0 0 1 2 2 2
  spline S155 degree 2 poles (-56.8536, -47.5704) (-57.9095, -47.5704) (-59.8176, -46.7738) (-60.5401, -46.0514) knots 0 0 0 1 2 2 2
  spline S156 degree 2 poles (-60.5401, -46.0514) (-61.2255, -45.3474) (-62.0592, -43.2726) (-62.0592, -42.124) knots 0 0 0 1 2 2 2
  spline S157 degree 2 poles (-62.0592, -42.124) (-62.0592, -40.3456) (-60.5586, -37.8262) (-58.9284, -37.1037) knots 0 0 0 1 2 2 2
  spline S158 degree 2 poles (-58.9284, -37.1037) (-57.4834, -36.4368) (-53.5561, -35.9367) (-51.2775, -35.807) knots 0 0 0 1 2 2 2
  line L108 (-51.2775, -35.807) -> (-51.2775, -35.2512)
  spline S159 degree 2 poles (-51.2775, -35.2512) (-51.2775, -34.2509) (-51.8889, -33.0097) (-52.4446, -32.6577) knots 0 0 0 1 2 2 2
  spline S160 degree 2 poles (-52.4446, -32.6577) (-53.0004, -32.3057) (-54.5935, -32.0834) (-55.4457, -32.0834) knots 0 0 0 1 2 2 2
  spline S161 degree 2 poles (-55.4457, -32.0834) (-56.446, -32.0834) (-59.1507, -32.6762) (-60.503, -33.2505) knots 0 0 0 1 2 2 2
  line L109 (-60.503, -33.2505) -> (-60.6698, -33.2505)
  line L110 (-60.6698, -33.2505) -> (-60.6698, -30.305)
  spline S162 degree 2 poles (-60.6698, -30.305) (-59.8732, -30.0827) (-56.8906, -29.527) (-55.4272, -29.527) knots 0 0 0 1 2 2 2
  spline S163 degree 2 poles (-55.4272, -29.527) (-53.6487, -29.527) (-51.222, -30.0827) (-50.2587, -30.8052) knots 0 0 0 1 2 2 2
  spline S164 degree 2 poles (-50.2587, -30.8052) (-49.3139, -31.5091) (-48.3876, -33.7507) (-48.3876, -35.3624) knots 0 0 0 1 2 2 2
  line L111 (-48.3876, -35.3624) -> (-48.3876, -47.0888)
  line L112 (-48.3876, -47.0888) -> (-51.2775, -47.0888)
  line L113 (-51.2775, -47.0888) -> (-51.2775, -45.2733)
  line L114 (-51.2775, -42.865) -> (-51.2775, -38.1041)
  spline S165 degree 2 poles (-51.2775, -38.1041) (-52.3149, -38.1967) (-55.4457, -38.5116) (-56.4275, -38.808) knots 0 0 0 1 2 2 2
  spline S166 degree 2 poles (-56.4275, -38.808) (-57.5761, -39.16) (-59.0766, -40.6235) (-59.0766, -41.9203) knots 0 0 0 1 2 2 2
  spline S167 degree 2 poles (-59.0766, -41.9203) (-59.0766, -43.4023) (-57.4093, -44.9028) (-55.8162, -44.9028) knots 0 0 0 1 2 2 2
  spline S168 degree 2 poles (-55.8162, -44.9028) (-54.4639, -44.9028) (-52.2408, -43.7357) (-51.2775, -42.865) knots 0 0 0 1 2 2 2
  line L115 (-35.3089, -25.9887) -> (-35.4571, -25.9887)
  spline S169 degree 2 poles (-35.4571, -25.9887) (-35.8461, -25.8405) (-37.2911, -25.5811) (-37.8653, -25.5811) knots 0 0 0 1 2 2 2
  spline S170 degree 2 poles (-37.8653, -25.5811) (-39.6808, -25.5811) (-41.2369, -27.2113) (-41.2369, -29.3602) knots 0 0 0 1 2 2 2
  line L116 (-41.2369, -29.3602) -> (-41.2369, -29.9345)
  line L117 (-41.2369, -29.9345) -> (-36.4574, -29.9345)
  line L118 (-36.4574, -29.9345) -> (-36.4574, -32.3243)
  line L119 (-36.4574, -32.3243) -> (-41.1443, -32.3243)
  line L120 (-41.1443, -32.3243) -> (-41.1443, -47.0888)
  line L121 (-41.1443, -47.0888) -> (-44.0342, -47.0888)
  line L122 (-44.0342, -47.0888) -> (-44.0342, -32.3243)
  line L123 (-44.0342, -32.3243) -> (-45.9793, -32.3243)
  line L124 (-45.9793, -32.3243) -> (-45.9793, -29.9345)
  line L125 (-45.9793, -29.9345) -> (-44.0342, -29.9345)
  line L126 (-44.0342, -29.9345) -> (-44.0342, -29.3602)
  spline S171 degree 2 poles (-44.0342, -29.3602) (-44.0342, -26.2851) (-41.0517, -23.0617) (-38.2729, -23.0617) knots 0 0 0 1 2 2 2
  spline S172 degree 2 poles (-38.2729, -23.0617) (-37.4763, -23.0617) (-35.9387, -23.2284) (-35.3089, -23.3396) knots 0 0 0 1 2 2 2
  line L127 (-35.3089, -23.3396) -> (-35.3089, -25.9887)
  spline S173 degree 2 poles (-28.4731, -47.4222) (-30.8258, -47.4222) (-33.4749, -44.7361) (-33.4749, -41.8276) knots 0 0 0 1 2 2 2
  line L128 (-33.4749, -41.8276) -> (-33.4749, -32.3243)
  line L129 (-33.4749, -32.3243) -> (-35.42, -32.3243)
  line L130 (-35.42, -32.3243) -> (-35.42, -29.9345)
  line L131 (-35.42, -29.9345) -> (-33.4749, -29.9345)
  line L132 (-33.4749, -29.9345) -> (-33.4749, -25.0068)
  line L133 (-33.4749, -25.0068) -> (-30.585, -25.0068)
  line L134 (-30.585, -25.0068) -> (-30.585, -29.9345)
  line L135 (-30.585, -29.9345) -> (-25.2683, -29.9345)
  line L136 (-25.2683, -29.9345) -> (-25.2683, -32.3243)
  line L137 (-25.2683, -32.3243) -> (-30.585, -32.3243)
  line L138 (-30.585, -32.3243) -> (-30.585, -40.4938)
  spline S174 degree 2 poles (-30.585, -40.4938) (-30.585, -41.7906) (-30.4923, -43.217) (-30.1774, -43.8284) knots 0 0 0 1 2 2 2
  spline S175 degree 2 poles (-30.1774, -43.8284) (-29.9181, -44.3656) (-28.751, -44.9028) (-27.7506, -44.9028) knots 0 0 0 1 2 2 2
  spline S176 degree 2 poles (-27.7506, -44.9028) (-27.0467, -44.9028) (-25.7314, -44.4767) (-25.435, -44.3471) knots 0 0 0 1 2 2 2
  line L139 (-25.435, -44.3471) -> (-25.2683, -44.3471)
  line L140 (-25.2683, -44.3471) -> (-25.2683, -46.9406)
  spline S177 degree 2 poles (-25.2683, -46.9406) (-26.0834, -47.1629) (-27.7506, -47.4222) (-28.4731, -47.4222) knots 0 0 0 1 2 2 2
  spline S178 degree 2 poles (-15.6908, -47.4778) (-19.8034, -47.4778) (-24.3235, -42.865) (-24.3235, -38.6043) knots 0 0 0 1 2 2 2
  spline S179 degree 2 poles (-24.3235, -38.6043) (-24.3235, -34.4176) (-19.933, -29.4529) (-16.3947, -29.4529) knots 0 0 0 1 2 2 2
  spline S180 degree 2 poles (-16.3947, -29.4529) (-14.8016, -29.4529) (-12.3377, -30.3791) (-11.43, -31.3609) knots 0 0 0 1 2 2 2
  spline S181 degree 2 poles (-11.43, -31.3609) (-10.5037, -32.3428) (-9.5219, -35.1771) (-9.5219, -37.2334) knots 0 0 0 1 2 2 2
  line L141 (-9.5219, -37.2334) -> (-9.5219, -38.808)
  line L142 (-9.5219, -38.808) -> (-21.3965, -38.808)
  spline S182 degree 2 poles (-21.3965, -38.808) (-21.3965, -41.7906) (-18.3954, -44.9584) (-15.7278, -44.9584) knots 0 0 0 1 2 2 2
  spline S183 degree 2 poles (-15.7278, -44.9584) (-14.783, -44.9584) (-12.9491, -44.5323) (-12.2081, -44.1989) knots 0 0 0 1 2 2 2
  spline S184 degree 2 poles (-12.2081, -44.1989) (-11.43, -43.8284) (-10.3555, -43.18) (-10.0036, -42.8836) knots 0 0 0 1 2 2 2
  line L143 (-10.0036, -42.8836) -> (-9.8368, -42.8836)
  line L144 (-9.8368, -42.8836) -> (-9.8368, -46.0328)
  spline S185 degree 2 poles (-9.8368, -46.0328) (-10.337, -46.2366) (-11.8561, -46.8294) (-12.4489, -46.9961) knots 0 0 0 1 2 2 2
  spline S186 degree 2 poles (-12.4489, -46.9961) (-13.2825, -47.237) (-14.6534, -47.4778) (-15.6908, -47.4778) knots 0 0 0 1 2 2 2
  spline S187 degree 2 poles (-12.3377, -36.6036) (-12.3748, -35.4365) (-12.8564, -33.7322) (-13.3196, -33.1579) knots 0 0 0 1 2 2 2
  spline S188 degree 2 poles (-13.3196, -33.1579) (-13.8197, -32.5095) (-15.3944, -31.8241) (-16.5615, -31.8241) knots 0 0 0 1 2 2 2
  spline S189 degree 2 poles (-16.5615, -31.8241) (-17.71, -31.8241) (-19.3217, -32.5095) (-19.9886, -33.1764) knots 0 0 0 1 2 2 2
  spline S190 degree 2 poles (-19.9886, -33.1764) (-20.637, -33.8618) (-21.3039, -35.5106) (-21.3965, -36.6036) knots 0 0 0 1 2 2 2
  line L145 (-21.3965, -36.6036) -> (-12.3377, -36.6036)
  line L146 (2.5009, -33.0282) -> (2.3527, -33.0282)
  spline S191 degree 2 poles (2.3527, -33.0282) (2.0192, -32.9356) (1.2968, -32.8985) (0.7966, -32.8985) knots 0 0 0 1 2 2 2
  spline S192 degree 2 poles (0.7966, -32.8985) (-0.3705, -32.8985) (-2.6676, -33.9174) (-3.705, -34.9178) knots 0 0 0 1 2 2 2
  line L147 (-3.705, -34.9178) -> (-3.705, -47.0888)
  line L148 (-3.705, -47.0888) -> (-6.5949, -47.0888)
  line L149 (-6.5949, -47.0888) -> (-6.5949, -29.9345)
  line L150 (-6.5949, -29.9345) -> (-3.705, -29.9345)
  line L151 (-3.705, -29.9345) -> (-3.705, -32.491)
  spline S193 degree 2 poles (-3.705, -32.491) (-2.1304, -31.0831) (0.2223, -29.9345) (1.3338, -29.9345) knots 0 0 0 1 2 2 2
  spline S194 degree 2 poles (1.3338, -29.9345) (1.7784, -29.9345) (2.223, -29.9716) (2.5009, -30.0271) knots 0 0 0 1 2 2 2
  line L152 (2.5009, -30.0271) -> (2.5009, -33.0282)
  spline S195 degree 2 poles (28.6584, -38.5116) (28.6584, -42.8465) (24.4902, -47.5704) (21.0075, -47.5704) knots 0 0 0 1 2 2 2
  spline S196 degree 2 poles (21.0075, -47.5704) (17.4321, -47.5704) (13.3381, -42.6983) (13.3381, -38.5116) knots 0 0 0 1 2 2 2
  spline S197 degree 2 poles (13.3381, -38.5116) (13.3381, -34.2138) (17.5618, -29.4529) (21.0075, -29.4529) knots 0 0 0 1 2 2 2
  spline S198 degree 2 poles (21.0075, -29.4529) (24.4902, -29.4529) (28.6584, -34.1953) (28.6584, -38.5116) knots 0 0 0 1 2 2 2
  spline S199 degree 2 poles (25.6758, -38.5116) (25.6758, -35.1771) (23.249, -31.9352) (21.0075, -31.9352) knots 0 0 0 1 2 2 2
  spline S200 degree 2 poles (21.0075, -31.9352) (18.7659, -31.9352) (16.3206, -35.1771) (16.3206, -38.5116) knots 0 0 0 1 2 2 2
  spline S201 degree 2 poles (16.3206, -38.5116) (16.3206, -41.7535) (18.7659, -45.0881) (21.0075, -45.0881) knots 0 0 0 1 2 2 2
  spline S202 degree 2 poles (21.0075, -45.0881) (23.2305, -45.0881) (25.6758, -41.8091) (25.6758, -38.5116) knots 0 0 0 1 2 2 2
  line L153 (45.0901, -47.0888) -> (42.2002, -47.0888)
  line L154 (42.2002, -47.0888) -> (42.2002, -37.3075)
  spline S203 degree 2 poles (42.2002, -37.3075) (42.2002, -36.1219) (41.9779, -34.0841) (41.6445, -33.4728) knots 0 0 0 1 2 2 2
  spline S204 degree 2 poles (41.6445, -33.4728) (41.2925, -32.8244) (40.0328, -32.1946) (38.9583, -32.1946) knots 0 0 0 1 2 2 2
  spline S205 degree 2 poles (38.9583, -32.1946) (37.8839, -32.1946) (35.6053, -33.3431) (34.5123, -34.2694) knots 0 0 0 1 2 2 2
  line L155 (34.5123, -34.2694) -> (34.5123, -47.0888)
  line L156 (34.5123, -47.0888) -> (31.6224, -47.0888)
  line L157 (31.6224, -47.0888) -> (31.6224, -29.9345)
  line L158 (31.6224, -29.9345) -> (34.5123, -29.9345)
  line L159 (34.5123, -29.9345) -> (34.5123, -31.8426)
  spline S206 degree 2 poles (34.5123, -31.8426) (35.8091, -30.6755) (38.31, -29.4529) (39.7179, -29.4529) knots 0 0 0 1 2 2 2
  spline S207 degree 2 poles (39.7179, -29.4529) (42.2373, -29.4529) (45.0901, -32.7874) (45.0901, -35.9552) knots 0 0 0 1 2 2 2
  line L160 (45.0901, -35.9552) -> (45.0901, -47.0888)
  spline S208 degree 2 poles (56.5942, -47.4778) (52.4817, -47.4778) (47.9615, -42.865) (47.9615, -38.6043) knots 0 0 0 1 2 2 2
  spline S209 degree 2 poles (47.9615, -38.6043) (47.9615, -34.4176) (52.352, -29.4529) (55.8903, -29.4529) knots 0 0 0 1 2 2 2
  spline S210 degree 2 poles (55.8903, -29.4529) (57.4835, -29.4529) (59.9473, -30.3791) (60.855, -31.3609) knots 0 0 0 1 2 2 2
  spline S211 degree 2 poles (60.855, -31.3609) (61.7813, -32.3428) (62.7631, -35.1771) (62.7631, -37.2334) knots 0 0 0 1 2 2 2
  line L161 (62.7631, -37.2334) -> (62.7631, -38.808)
  line L162 (62.7631, -38.808) -> (50.8885, -38.808)
  spline S212 degree 2 poles (50.8885, -38.808) (50.8885, -41.7906) (53.8896, -44.9584) (56.5572, -44.9584) knots 0 0 0 1 2 2 2
  spline S213 degree 2 poles (56.5572, -44.9584) (57.502, -44.9584) (59.336, -44.5323) (60.077, -44.1989) knots 0 0 0 1 2 2 2
  spline S214 degree 2 poles (60.077, -44.1989) (60.855, -43.8284) (61.9295, -43.18) (62.2815, -42.8836) knots 0 0 0 1 2 2 2
  line L163 (62.2815, -42.8836) -> (62.4482, -42.8836)
  line L164 (62.4482, -42.8836) -> (62.4482, -46.0328)
  spline S215 degree 2 poles (62.4482, -46.0328) (61.948, -46.2366) (60.4289, -46.8294) (59.8361, -46.9961) knots 0 0 0 1 2 2 2
  spline S216 degree 2 poles (59.8361, -46.9961) (59.0025, -47.237) (57.6317, -47.4778) (56.5942, -47.4778) knots 0 0 0 1 2 2 2
  spline S217 degree 2 poles (59.9473, -36.6036) (59.9102, -35.4365) (59.4286, -33.7322) (58.9655, -33.1579) knots 0 0 0 1 2 2 2
  spline S218 degree 2 poles (58.9655, -33.1579) (58.4653, -32.5095) (56.8906, -31.8241) (55.7236, -31.8241) knots 0 0 0 1 2 2 2
  spline S219 degree 2 poles (55.7236, -31.8241) (54.575, -31.8241) (52.9633, -32.5095) (52.2964, -33.1764) knots 0 0 0 1 2 2 2
  spline S220 degree 2 poles (52.2964, -33.1764) (51.648, -33.8618) (50.9811, -35.5106) (50.8885, -36.6036) knots 0 0 0 1 2 2 2
  line L165 (50.8885, -36.6036) -> (59.9473, -36.6036)
  line L166 (-26.3057, -84.5054) -> (-26.3057, -74.5759)
  spline S221 degree 2 poles (-26.3057, -74.5759) (-26.3057, -73.3903) (-26.4909, -71.3711) (-26.7873, -70.8153) knots 0 0 0 1 2 2 2
  spline S222 degree 2 poles (-26.7873, -70.8153) (-27.0837, -70.204) (-28.2138, -69.6112) (-29.1956, -69.6112) knots 0 0 0 1 2 2 2
  spline S223 degree 2 poles (-29.1956, -69.6112) (-30.0848, -69.6112) (-32.1226, -70.7042) (-33.197, -71.7416) knots 0 0 0 1 2 2 2
  spline S224 degree 2 poles (-33.197, -71.7416) (-33.1785, -72.0009) (-33.1414, -72.7234) (-33.1414, -73.2051) knots 0 0 0 1 2 2 2
  line L167 (-33.1414, -73.2051) -> (-33.1414, -84.5054)
  line L168 (-33.1414, -84.5054) -> (-36.0314, -84.5054)
  line L169 (-36.0314, -84.5054) -> (-36.0314, -74.5759)
  spline S225 degree 2 poles (-36.0314, -74.5759) (-36.0314, -73.3903) (-36.2166, -71.3711) (-36.513, -70.8153) knots 0 0 0 1 2 2 2
  spline S226 degree 2 poles (-36.513, -70.8153) (-36.8094, -70.204) (-37.9394, -69.6112) (-38.9213, -69.6112) knots 0 0 0 1 2 2 2
  spline S227 degree 2 poles (-38.9213, -69.6112) (-39.8475, -69.6112) (-41.9038, -70.7783) (-42.8671, -71.686) knots 0 0 0 1 2 2 2
  line L170 (-42.8671, -71.686) -> (-42.8671, -84.5054)
  line L171 (-42.8671, -84.5054) -> (-45.7571, -84.5054)
  line L172 (-45.7571, -84.5054) -> (-45.7571, -67.3511)
  line L173 (-45.7571, -67.3511) -> (-42.8671, -67.3511)
  line L174 (-42.8671, -67.3511) -> (-42.8671, -69.2407)
  spline S228 degree 2 poles (-42.8671, -69.2407) (-41.7371, -68.1107) (-39.5141, -66.8695) (-38.1803, -66.8695) knots 0 0 0 1 2 2 2
  spline S229 degree 2 poles (-38.1803, -66.8695) (-36.6612, -66.8695) (-34.3085, -68.2589) (-33.6972, -69.8335) knots 0 0 0 1 2 2 2
  spline S230 degree 2 poles (-33.6972, -69.8335) (-32.3819, -68.37) (-29.8995, -66.8695) (-28.4546, -66.8695) knots 0 0 0 1 2 2 2
  spline S231 degree 2 poles (-28.4546, -66.8695) (-27.3431, -66.8695) (-25.5276, -67.5549) (-24.8607, -68.333) knots 0 0 0 1 2 2 2
  spline S232 degree 2 poles (-24.8607, -68.333) (-24.1753, -69.111) (-23.4158, -71.4452) (-23.4158, -73.2051) knots 0 0 0 1 2 2 2
  line L175 (-23.4158, -73.2051) -> (-23.4158, -84.5054)
  line L176 (-23.4158, -84.5054) -> (-26.3057, -84.5054)
  line L177 (-16.4133, -84.5054) -> (-19.3032, -84.5054)
  line L178 (-19.3032, -84.5054) -> (-19.3032, -67.3511)
  line L179 (-19.3032, -67.3511) -> (-16.4133, -67.3511)
  line L180 (-16.4133, -67.3511) -> (-16.4133, -84.5054)
  line L181 (-16.2095, -64.4983) -> (-19.4884, -64.4983)
  line L182 (-19.4884, -64.4983) -> (-19.4884, -61.4972)
  line L183 (-19.4884, -61.4972) -> (-16.2095, -61.4972)
  line L184 (-16.2095, -61.4972) -> (-16.2095, -64.4983)
  line L185 (1.2968, -84.5054) -> (-1.5932, -84.5054)
  line L186 (-1.5932, -84.5054) -> (-1.5932, -74.7241)
  spline S233 degree 2 poles (-1.5932, -74.7241) (-1.5932, -73.5385) (-1.8155, -71.5008) (-2.1489, -70.8894) knots 0 0 0 1 2 2 2
  spline S234 degree 2 poles (-2.1489, -70.8894) (-2.5009, -70.2411) (-3.7606, -69.6112) (-4.8351, -69.6112) knots 0 0 0 1 2 2 2
  spline S235 degree 2 poles (-4.8351, -69.6112) (-5.9095, -69.6112) (-8.1881, -70.7598) (-9.2811, -71.686) knots 0 0 0 1 2 2 2
  line L187 (-9.2811, -71.686) -> (-9.2811, -84.5054)
  line L188 (-9.2811, -84.5054) -> (-12.171, -84.5054)
  line L189 (-12.171, -84.5054) -> (-12.171, -67.3511)
  line L190 (-12.171, -67.3511) -> (-9.2811, -67.3511)
  line L191 (-9.2811, -67.3511) -> (-9.2811, -69.2592)
  spline S236 degree 2 poles (-9.2811, -69.2592) (-7.9843, -68.0921) (-5.4834, -66.8695) (-4.0755, -66.8695) knots 0 0 0 1 2 2 2
  spline S237 degree 2 poles (-4.0755, -66.8695) (-1.5561, -66.8695) (1.2968, -70.204) (1.2968, -73.3718) knots 0 0 0 1 2 2 2
  line L192 (1.2968, -73.3718) -> (1.2968, -84.5054)
  line L193 (18.6918, -84.5054) -> (15.8019, -84.5054)
  line L194 (15.8019, -84.5054) -> (15.8019, -82.6158)
  spline S238 degree 2 poles (15.8019, -82.6158) (14.4681, -83.7829) (12.0784, -84.987) (10.5964, -84.987) knots 0 0 0 1 2 2 2
  spline S239 degree 2 poles (10.5964, -84.987) (9.4849, -84.987) (7.5027, -84.246) (6.7802, -83.4495) knots 0 0 0 1 2 2 2
  spline S240 degree 2 poles (6.7802, -83.4495) (6.0392, -82.6529) (5.2241, -80.2261) (5.2241, -78.4847) knots 0 0 0 1 2 2 2
  line L195 (5.2241, -78.4847) -> (5.2241, -67.3511)
  line L196 (5.2241, -67.3511) -> (8.114, -67.3511)
  line L197 (8.114, -67.3511) -> (8.114, -77.1324)
  spline S241 degree 2 poles (8.114, -77.1324) (8.114, -78.5033) (8.3178, -80.3002) (8.6698, -80.9671) knots 0 0 0 1 2 2 2
  spline S242 degree 2 poles (8.6698, -80.9671) (9.0217, -81.634) (10.2259, -82.2453) (11.3559, -82.2453) knots 0 0 0 1 2 2 2
  spline S243 degree 2 poles (11.3559, -82.2453) (12.4118, -82.2453) (14.8016, -81.0412) (15.8019, -80.1705) knots 0 0 0 1 2 2 2
  line L198 (15.8019, -80.1705) -> (15.8019, -67.3511)
  line L199 (15.8019, -67.3511) -> (18.6918, -67.3511)
  line L200 (18.6918, -67.3511) -> (18.6918, -84.5054)
  spline S244 degree 2 poles (28.0656, -84.8388) (25.7129, -84.8388) (23.0638, -82.1527) (23.0638, -79.2443) knots 0 0 0 1 2 2 2
  line L201 (23.0638, -79.2443) -> (23.0638, -69.7409)
  line L202 (23.0638, -69.7409) -> (21.1186, -69.7409)
  line L203 (21.1186, -69.7409) -> (21.1186, -67.3511)
  line L204 (21.1186, -67.3511) -> (23.0638, -67.3511)
  line L205 (23.0638, -67.3511) -> (23.0638, -62.4235)
  line L206 (23.0638, -62.4235) -> (25.9537, -62.4235)
  line L207 (25.9537, -62.4235) -> (25.9537, -67.3511)
  line L208 (25.9537, -67.3511) -> (31.2704, -67.3511)
  line L209 (31.2704, -67.3511) -> (31.2704, -69.7409)
  line L210 (31.2704, -69.7409) -> (25.9537, -69.7409)
  line L211 (25.9537, -69.7409) -> (25.9537, -77.9105)
  spline S245 degree 2 poles (25.9537, -77.9105) (25.9537, -79.2072) (26.0463, -80.6336) (26.3612, -81.245) knots 0 0 0 1 2 2 2
  spline S246 degree 2 poles (26.3612, -81.245) (26.6206, -81.7822) (27.7877, -82.3194) (28.788, -82.3194) knots 0 0 0 1 2 2 2
  spline S247 degree 2 poles (28.788, -82.3194) (29.492, -82.3194) (30.8073, -81.8934) (31.1037, -81.7637) knots 0 0 0 1 2 2 2
  line L212 (31.1037, -81.7637) -> (31.2704, -81.7637)
  line L213 (31.2704, -81.7637) -> (31.2704, -84.3572)
  spline S248 degree 2 poles (31.2704, -84.3572) (30.4553, -84.5795) (28.788, -84.8388) (28.0656, -84.8388) knots 0 0 0 1 2 2 2
  spline S249 degree 2 poles (40.8479, -84.8944) (36.7353, -84.8944) (32.2152, -80.2817) (32.2152, -76.0209) knots 0 0 0 1 2 2 2
  spline S250 degree 2 poles (32.2152, -76.0209) (32.2152, -71.8342) (36.6056, -66.8695) (40.1439, -66.8695) knots 0 0 0 1 2 2 2
  spline S251 degree 2 poles (40.1439, -66.8695) (41.7371, -66.8695) (44.2009, -67.7957) (45.1087, -68.7776) knots 0 0 0 1 2 2 2
  spline S252 degree 2 poles (45.1087, -68.7776) (46.0349, -69.7594) (47.0168, -72.5937) (47.0168, -74.65) knots 0 0 0 1 2 2 2
  line L214 (47.0168, -74.65) -> (47.0168, -76.2247)
  line L215 (47.0168, -76.2247) -> (35.1422, -76.2247)
  spline S253 degree 2 poles (35.1422, -76.2247) (35.1422, -79.2072) (38.1432, -82.375) (40.8108, -82.375) knots 0 0 0 1 2 2 2
  spline S254 degree 2 poles (40.8108, -82.375) (41.7556, -82.375) (43.5896, -81.9489) (44.3306, -81.6155) knots 0 0 0 1 2 2 2
  spline S255 degree 2 poles (44.3306, -81.6155) (45.1087, -81.245) (46.1831, -80.5966) (46.5351, -80.3002) knots 0 0 0 1 2 2 2
  line L216 (46.5351, -80.3002) -> (46.7018, -80.3002)
  line L217 (46.7018, -80.3002) -> (46.7018, -83.4495)
  spline S256 degree 2 poles (46.7018, -83.4495) (46.2017, -83.6532) (44.6826, -84.246) (44.0898, -84.4128) knots 0 0 0 1 2 2 2
  spline S257 degree 2 poles (44.0898, -84.4128) (43.2562, -84.6536) (41.8853, -84.8944) (40.8479, -84.8944) knots 0 0 0 1 2 2 2
  spline S258 degree 2 poles (44.2009, -74.0202) (44.1639, -72.8531) (43.6822, -71.1488) (43.2191, -70.5745) knots 0 0 0 1 2 2 2
  spline S259 degree 2 poles (43.2191, -70.5745) (42.7189, -69.9261) (41.1443, -69.2407) (39.9772, -69.2407) knots 0 0 0 1 2 2 2
  spline S260 degree 2 poles (39.9772, -69.2407) (38.8287, -69.2407) (37.217, -69.9261) (36.5501, -70.593) knots 0 0 0 1 2 2 2
  spline S261 degree 2 poles (36.5501, -70.593) (35.9017, -71.2785) (35.2348, -72.9272) (35.1422, -74.0202) knots 0 0 0 1 2 2 2
  line L218 (35.1422, -74.0202) -> (44.2009, -74.0202)
  point P0 (0, 0)
  dimension "d13" = 177.8
  dimension "d16" = 34.29
  constraints: 2 end point, 2 horizontal, 2 point on line
  measures "d16" distance between parallel lines of L1 L3
emboss "Emboss2" sketch "Sketch5" operation cut depth 2.54 direction (0, 0, -1)
sketch "Sketch6" plane through (0, 0, 0) normal (0, 0, 1) x (1, 0, 0)
  line L0 (-76.2, -88.9) -> (76.2, -88.9) construction
  line L1 (76.2, -88.9) -> (76.2, 88.9) construction
  line L2 (76.2, 88.9) -> (-76.2, 88.9) construction
  line L3 (-76.2, 88.9) -> (-76.2, -88.9) construction
  line L4 (-76.2, -88.9) -> (76.2, 88.9) construction
  line L5 (76.2, -88.9) -> (-76.2, 88.9) construction
  point P0 (0, 0)
  dimension "d19" = 177.8
  dimension "d20" = 152.4
  constraints: 12 end point, 4 coincident, 2 midpoint, 2 parallel, 1 horizontal, 1 perpendicular
  measures "d19" distance of L2.end L0.start
  measures "d20" distance of L0.start L0.end
hole "Hole1" at (-76.2, 88.9, 0) at (76.2, 88.9, 0) at (76.2, -88.9, 0) at (-76.2, -88.9, 0) direction (0, 0, -1) diameter 6.35 end through all
body "Solid2"
